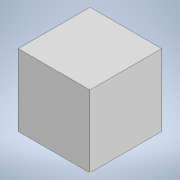
# Autodesk Inventor part: pawn-2
Saved by Autodesk Inventor 2021 (Build 250183000, 183)
## iProperties
Created: 2021-01-10
Part Number: pawn-2
Material: Generic
Document SubType Name: Modeling
Designer: Luke Kamols
Density: 1 g/cm^3
Appearance: Default
Author: Luke Kamols
Autodesk Inventor part; units mm, degrees
ref_plane "YZ Plane" through (0, 0, 0) normal (1, 0, 0) x (0, 1, 0)
ref_plane "XZ Plane" through (0, 0, 0) normal (0, 1, 0) x (-1, 0, 0)
ref_plane "XY Plane" through (0, 0, 0) normal (0, 0, 1) x (1, 0, 0)
sketch "Sketch1" plane through (0, 0, 0) normal (0, 1, 0) x (-1, 0, 0)
  point P0 (0, 0)
sketch "Sketch2" plane through (0, 0, 0) normal (0, 1, 0) x (-1, 0, 0)
  line L0 (0, 0) -> (16, 0)
  line L1 (16, 0) -> (16, -16)
  line L2 (16, -16) -> (0, -16)
  line L3 (0, -16) -> (0, 0)
  line L4 (0, 0) -> (0, -8)
  dimension "d1" = 16
  dimension "d2" = 16
  constraints: 10 end point, 2 parallel, 1 horizontal, 1 midpoint, 1 perpendicular
  measures "d1" distance of L1.end L2.end
  measures "d2" distance of L0.end L1.end
extrude "Extrusion1" add sketch "Sketch2" along normal blind 16
sketch "Sketch3" plane through (0, 0, 0) normal (0, -1, 0) x (1, 0, 0)
  line L0 (-16, 0) -> (0, 0) projected
  line L1 (-16, -16) -> (-16, 0) projected
  line L2 (0, 0) -> (0, -16) projected
  line L3 (-16, -8) -> (0, -8)
  line L4 (-16, -8) -> (-16, -9.8)
  line L5 (0, -16) -> (0, -14.2)
  line L6 (0, -14.2) -> (-16, -9.8)
  line L7 (-8, -12) -> (-1.7327, -13.7235)
  line L8 (-1.7327, -13.7235) -> (-1.2135, -12)
  line L9 (-1.2135, -12) -> (-13.7482, -8.553)
  line L10 (-13.7482, -8.553) -> (-14.7865, -12)
  line L11 (-14.7865, -12) -> (-2.3425, -15.7481)
  line L12 (-2.3425, -15.7481) -> (-1.7327, -13.7235)
  line L13 (-16, -8) -> (-16, -6.2)
  line L14 (0, 0) -> (0, -1.8)
  line L15 (0, -1.8) -> (-16, -6.2)
  line L16 (-8, -4) -> (-14.2673, -5.7235)
  line L17 (-14.2673, -5.7235) -> (-13.7901, -7.4591)
  line L18 (-13.7901, -7.4591) -> (-1.2554, -4.0121)
  line L19 (-13.7901, -7.4591) -> (-14.7446, -3.9879)
  line L20 (-14.7446, -3.9879) -> (-2.2099, -0.5409)
  line L21 (-2.2099, -0.5409) -> (-1.2554, -4.0121)
  dimension "d28" = 1.8
  dimension "d31" = 1.8
  dimension "d32" = 13
  dimension "d33" = 3.6
  dimension "d34" = 1.8
  dimension "d35" = 1.8
  dimension "d37" = 1.8
  dimension "d38" = 13
  dimension "d42" = 3.6
  dimension "d43" = 13
  constraints: 38 end point, 8 point on line, 5 perpendicular, 4 midpoint, 2 parallel
  measures "d28" distance of L3.start L4.end
  measures "d31" distance of L7.end L8.end
  measures "d32" distance of L8.end L9.end
  measures "d33" distance of L9.end L10.end
  measures "d34" distance of L3.start L13.end
  measures "d35" distance of L0.end L14.end
  measures "d37" distance of L16.end L17.end
  measures "d38" distance of L17.end L18.end
  measures "d42" distance of L17.end L19.end
  measures "d43" distance of L19.end L20.end
extrude "Extrusion2" cut sketch "Sketch3" against normal blind 13 contours L19 L20 L21 L15 | L15 L21 L18 L17 | L10 L9 L8 L6 | L6 L12 L11 L10
body "Solid1"
